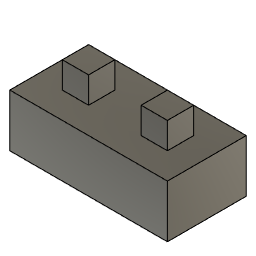
2x1Block (Autodesk Fusion 360 design; units mm, degrees)
Autodesk Fusion 360 part; units mm, degrees
sketch "Sketch1" plane through (0, 0, 0) normal (0, 0, 1) x (1, 0, 0)
  line L0 (0, 0) -> (-30, 0)
  line L1 (-30, 0) -> (-30, 15)
  line L2 (-30, 15) -> (0, 15)
  line L3 (0, 15) -> (0, 0)
  line L4 (-15, 0) -> (-15, 15)
  line L5 (-25, 10) -> (-20, 10)
  line L6 (-20, 10) -> (-20, 5)
  line L7 (-20, 5) -> (-25, 5)
  line L8 (-25, 5) -> (-25, 10)
  line L9 (-10, 10) -> (-5, 10)
  line L10 (-5, 10) -> (-5, 5)
  line L11 (-5, 5) -> (-10, 5)
  line L12 (-10, 5) -> (-10, 10)
  line L13 (-25.175, 10.175) -> (-19.825, 10.175)
  line L14 (-19.825, 10.175) -> (-19.825, 4.825)
  line L15 (-19.825, 4.825) -> (-25.175, 4.825)
  line L16 (-25.175, 4.825) -> (-25.175, 10.175)
  line L17 (-10.175, 10.175) -> (-4.825, 10.175)
  line L18 (-4.825, 10.175) -> (-4.825, 4.825)
  line L19 (-4.825, 4.825) -> (-10.175, 4.825)
  line L20 (-10.175, 4.825) -> (-10.175, 10.175)
  dimension "d1" = 30
  dimension "d2" = 15
  dimension "d7" = -0.175
  dimension "d8" = -0.175
  constraint horizontal L0
  constraint vertical L1
  constraint horizontal L2
  constraint vertical L3
  constraint coincident L0.start L3.end
  constraint midpoint L0 L4.start
  constraint midpoint L2 L4.end
  constraint horizontal L5
  constraint vertical L6
  constraint horizontal L7
  constraint vertical L8
  constraint horizontal L9
  constraint vertical L10
  constraint horizontal L11
  constraint vertical L12
  measures "d1" distance of L0.start L0.end
  measures "d2" distance of L0.start L2.end
extrude "Extrude1" add sketch "Sketch1" along normal blind 10 contours L0 L2 L3 L4 | L0 L1 L2 L4 | L13 L14 L15 L16 | L17 L18 L19 L20
extrude "Extrude2" add sketch "Sketch1" along normal blind 15 contours L5 L6 L7 L8 | L9 L10 L11 L12
extrude "Extrude3" cut sketch "Sketch1" along normal blind 5.175 contours L5 L6 L7 L8 | L9 L10 L11 L12 | L13 L14 L15 L16 | L17 L18 L19 L20
